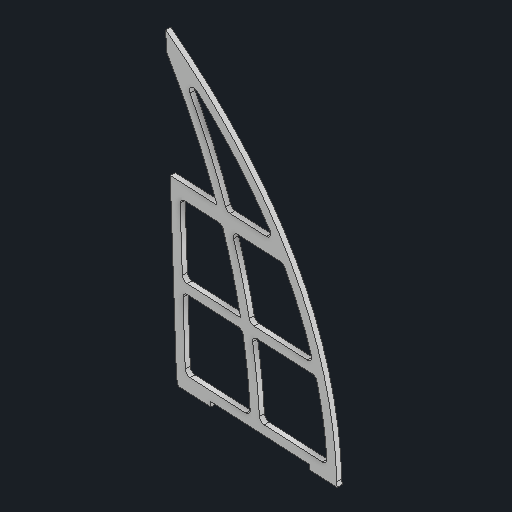
# Autodesk Inventor part: sponson_spanner_side
Saved by Autodesk Inventor 2023 (Build 270158030, 158C)
## iProperties
Created: 2022-03-22
Part Number: sponson_spanner_side
Material: Generic
Document SubType Name: Modeling
Designer: kardo
Density: 1 g/cm^3
Appearance: Default
Author: kardo
Autodesk Inventor part; units mm, degrees
ref_plane "YZ Plane" through (0, 0, 0) normal (1, 0, 0) x (0, 1, 0)
ref_plane "XZ Plane" through (0, 0, 0) normal (0, 1, 0) x (-1, 0, 0)
ref_plane "XY Plane" through (0, 0, 0) normal (0, 0, 1) x (1, 0, 0)
derived "surface_body.ipt"
sketch "sk_rail_sponson_side" plane through (81.12, 255, 36.448) normal (0.0461938, 0.0348622, -0.998324) x (0.2816917, -0.9592867, -0.0204648)
  line L0 (265.8225, 0) -> (150.1079, -34.011)
  spline S0 degree 2 poles (150.1079, -34.011) (71.6005, -57.0859) (0, 0) knots 0 0 0 1 1 1
  point P0 (222.5132, 151.1878)
ref_plane "plane_tunnel_right" through (81.12, 0, 0) normal (1, 0, 0) x (0, 1, 0)
ref_plane "plane_sponson_side" through (81.12, 255, 36.448) normal (0.0461938, 0.0348622, -0.998324) x (0.2816917, -0.9592867, -0.0204648)
sketch "sk_rail_sponson_tunnel" plane through (81.12, 0, 0) normal (1, 0, 0) x (0, 1, 0)
  line L0 (0, 0) -> (122.4, 8.559)
  line L1 (112.6461, 148.0459) -> (139.8617, -241.1549) construction
  spline S0 degree 2 poles (122.4, 8.559) (190.3044, 13.3074) (255, 36.448) knots 0 0 0 1 1 1
sketch "sk_rail_sponson_bottom" plane through (126.048, 0, 0) normal (0.3820078, -0.0644661, 0.9219079) x (-0.1718217, 0.9752166, 0.139391)
  line L0 (120.5596, -22.8124) -> (0, 0)
  line L1 (389.238, -73.6522) -> (-473.5511, 89.606) construction
  line L2 (163.9663, 206.5842) -> (90.6689, -180.7791) construction
  spline S0 degree 2 poles (120.5596, -22.8124) (192.7887, -36.4798) (261.4804, 0) knots 0 0 0 1 1 1
  point P0 (21.6578, 114.4574)
sketch "sk_rail_top_tunnel" plane through (81.12, 0, 0) normal (1, 0, 0) x (0, 1, 0)
  line L0 (255, 107.6209) -> (255, -224.5198) construction
  line L1 (0, 107.6209) -> (0, -224.5198) construction
  line L2 (-345, 107.6209) -> (-345, -224.5198) construction
  line L3 (-345, 0) -> (0, 0) construction
  line L4 (-172.5, 48.8998) -> (-172.5, 0) construction
  line L5 (0, 52.89) -> (37.026, 52.89) construction
  line L6 (37.026, 52.89) -> (80.784, 47.0555) construction
  line L7 (80.784, 47.0555) -> (112.2, 37.536) construction
  line L8 (112.2, 107.6209) -> (112.2, -224.5198) construction
  line L9 (0, 52.89) -> (255, 52.89) construction
  line L10 (-469.9272, 0) -> (379.2584, 0) construction
  spline S0 degree 3 poles (0, 52.89) (92.8353, 52.89) (195.0311, 49.5089) (255, 36.448) knots 0 0 0 0 1 1 1 1
  spline S1 degree 3 poles (0, 52.89) (37.026, 52.89) (80.784, 47.0555) (112.2, 37.536) knots 1 1 1 1 2 2 2 2
  spline S2 degree 4 poles (-345, 37.4554) (-258.8682, 45.1562) (-172.5926, 49.7838) (-86.3161, 52.89) (0, 52.89) knots 0 0 0 0 0 1 1 1 1 1
  point P0 (153, 48.7795)
  point P1 (112.2, 28.832)
  point P2 (-230.0001, 45.8702)
  point P3 (-114.9999, 51.0173)
sketch "sk_section_sponson_break" plane through (0, 122.4, 8.559) normal (0, 0.9975641, 0.0697565) x (-1, 0, 0)
  line L0 (-273.529, -60.9623) -> (62.2867, 77.8495) construction
  line L1 (-81.12, -262.9814) -> (-81.12, 151.9167) construction
  arc A0 (-81.12, 42.1186) -> (-156, 26.7233) centre (-71.3066, -195.4114) ccw construction
  arc A1 (-54.6, 54.2675) -> (-156, 30.9325) centre (-53.2768, -183.4615) ccw construction
  spline S0 degree 2 poles (-54.6, 54.2675) (-107.2974, 54.2675) (-156, 30.9325) knots 0 0 0 1 1 1
  spline S1 degree 2 poles (-156, 26.7233) (-120.0524, 40.429) (-81.12, 42.1186) knots 0 0 0 1 1 1
  point P0 (0, 0)
ref_plane "plane_sponson_break" through (0, 122.4, 8.559) normal (0, 0.9975641, 0.0697565) x (-1, 0, 0)
derived "parameters_frame.ipt"
derived "stencil_frame.ipt"
sketch "sk_joint_locations" plane through (81.12, 0, 0) normal (1, 0, 0) x (0, 1, 0)
  line L0 (0, 0) -> (122.4, 8.559) construction
  line L1 (36.465, 28.832) -> (112.2, 28.832) construction
  arc A0 (36.465, 28.832) -> (11.22, 28.376) centre (36.465, -670.197) ccw construction
  line L2 (-241.5001, 19.2432) -> (11.22, 28.376) construction
  line L3 (-345, 16.32) -> (-262.2001, 18.586) construction
  arc A1 (-262.2001, 18.586) -> (-241.5001, 19.2432) centre (-326.8578, 2381.2399) ccw construction
  line L4 (-95.1358, 3119.4657) -> (254.2444, -1876.9042) construction
  line L5 (-230.0001, 3089.1136) -> (-230.0001, -1866.0023) construction
  line L6 (-114.9999, 3089.1136) -> (-114.9999, -1866.0023) construction
  line L7 (-345, 3089.1136) -> (-345, -1866.0023) construction
  line L8 (0, 3089.1136) -> (0, -1866.0023) construction
  line L9 (516.4305, 45.5774) -> (-594.5903, 6.7797) construction
  line L10 (-657.7604, -27.3784) -> (621.8174, 62.0984) construction
  line L11 (193.4506, 30.2962) -> (193.1714, 38.2913) construction
  line L12 (201.1621, 36.7028) -> (201.7215, 28.7028) construction
  line L13 (0, 14.96) -> (121.9304, 15.2746) construction
  line L14 (-230.0001, 45.8702) -> (-230.0001, 19.6588) construction
  line L15 (-345, 37.4554) -> (-345, 16.32) construction
  line L16 (-114.9999, 51.0173) -> (-114.9999, 23.8147) construction
  line L17 (0, 52.89) -> (0, 27.9705) construction
  line L18 (119.462, 50.575) -> (119.9556, 43.5149) construction
  line L19 (120.4493, 36.4549) -> (119.9556, 43.5149) construction
  line L20 (120.4493, 36.4549) -> (120.943, 29.3948) construction
  line L21 (120.943, 29.3948) -> (121.4367, 22.3347) construction
  line L22 (121.4367, 22.3347) -> (121.9304, 15.2746) construction
  line L23 (0, 14.96) -> (0, 0) construction
  line L24 (112.2, 37.536) -> (112.2, 28.832) construction
  line L25 (112.2, 35.548) -> (112.2, 30.82) construction
  spline S0 degree 4 poles (-345, 37.4554) (-258.8682, 45.1562) (-172.5926, 49.7838) (-86.3161, 52.89) (0, 52.89) knots 0 0 0 0 0 1 1 1 1 1
  spline S1 degree 3 poles (0, 52.89) (92.8353, 52.89) (195.0311, 49.5089) (255, 36.448) knots 0 0 0 0 1 1 1 1
  spline S2 degree 2 poles (122.4, 8.559) (190.3044, 13.3074) (255, 36.448) knots 0 0 0 1 1 1
  point P0 (-95.1358, 3119.4657)
  point P1 (254.2444, -1876.9042)
  point P2 (193.311, 34.2938)
  point P3 (201.4418, 32.7028)
  point P4 (134.9575, 11.3411)
  point P5 (-345, 26.8877)
  point P6 (-230.0001, 32.7645)
  point P7 (-114.9999, 37.416)
  point P8 (0, 40.4303)
  point P9 (112.2, 33.184)
sketch "sk_spanner_joints_locations" plane through (0, 122.4, 8.559) normal (0, 0.9975641, 0.0697565) x (-1, 0, 0)
  line L0 (300.9234, 5.5808) -> (-420.7494, 38.9736) construction
  line L1 (-923.3057, -329.5522) -> (1264.6454, 574.8532) construction
  line L2 (-84.7099, 23.4246) -> (-83.6779, 17.514) construction
  line L3 (-84.7099, 23.4246) -> (-70.9223, 22.7866) construction
  line L4 (-83.6779, 17.514) -> (-70.9223, 22.7866) construction
  point P0 (0, 0)
  point P1 (-126.048, 0)
  point P2 (-156, 26.7233)
  point P3 (-141.742, 26.0635)
  point P4 (-98.9679, 24.0843)
  point P5 (-94.2704, 13.1355)
  point P6 (-115.4555, 4.3785)
ref_plane "plane_stringer_outer" through (84.12, 0, 0) normal (1, 0, 0) x (0, 1, 0)
sketch "sk_corner_offset" plane through (0, 122.4, 8.559) normal (0, 0.9975641, 0.0697565) x (-1, 0, 0)
  spline S0 degree 2 poles (-156, 26.7233) (-120.0524, 40.429) (-81.12, 42.1186) knots 0 0 0 1 1 1 construction
  line L0 (-156, 26.7233) -> (-126.048, 0) construction
  line L1 (-153.7218, 26.2989) -> (-125.2491, 0.8954) construction
  line L2 (-125.2491, 0.8954) -> (-126.048, 0) construction
  spline S1 degree 5 poles (-153.7218, 26.2988) (-139.7718, 31.4859) (-125.4179, 35.5876) (-110.7581, 38.5194) (-95.9372, 40.2742) (-81.068, 40.9197) knots 0 0 0 0 0 0 1 1 1 1 1 1 construction
  point P0 (0, 0)
  dimension "d9" = 1.2
  dimension "d10" = 1.2
  constraints: 6 end point, 1 coincident, 1 parallel, 1 perpendicular, 3 other
  measures "d10" distance between parallel lines of L1 L0
sketch "sk_tip_offset" plane through (81.12, 0, 0) normal (1, 0, 0) x (0, 1, 0)
  spline S0 degree 3 poles (0, 52.89) (92.8353, 52.89) (195.0311, 49.5089) (255, 36.448) knots 0 0 0 0 1 1 1 1 construction
  spline S1 degree 2 poles (122.4, 8.559) (190.3044, 13.3074) (255, 36.448) knots 0 0 0 1 1 1 construction
  spline S2 degree 5 poles (0, 51.69) (14.1108, 51.69) (28.2217, 51.6249) (42.3321, 51.4877) (70.2924, 51.0558) (98.2445, 50.2552) (112.0882, 49.7555) (138.5614, 48.5709) (165.0044, 46.8436) (177.6143, 45.8726) (199.84, 43.8477) (221.9828, 41.066) (231.553, 39.6839) (241.0942, 38.0879) (250.5671, 36.1558) knots 0 0 0 0 0 0 0.280662 0.280662 0.280662 0.556179 0.556179 0.556179 0.807705 0.807705 0.807705 1 1 1 1 1 1 construction
  spline S3 degree 5 poles (122.3163, 9.7561) (148.5177, 11.5885) (174.5986, 15.1479) (200.4027, 20.4751) (225.7629, 27.5171) (250.5671, 36.1559) knots 0 0 0 0 0 0 1 1 1 1 1 1 construction
  point P0 (0, 0)
  dimension "d7" = 1.2
  dimension "d8" = 1.2
  constraints: 1 coincident, 6 other
sketch "sk_sponson_spanner_side_base" plane through (81.12, 255, 36.448) normal (0.0461938, 0.0348622, -0.998324) x (0.2816917, -0.9592867, -0.0204648)
  spline S0 degree 2 poles (150.1079, -34.011) (71.6005, -57.0859) (0, 0) knots 0 0 0 1 1 1 construction
  line L0 (129.8727, 34.4266) -> (129.7052, 34.9929)
  line L1 (133.9197, 20.7391) -> (146.0609, -20.3235)
  line L2 (146.0609, -20.3235) -> (147.9788, -19.7564)
  line L3 (147.9788, -19.7564) -> (151.3759, -31.2458)
  line L4 (133.9197, 20.7391) -> (135.8376, 21.3061)
  line L5 (135.8376, 21.3061) -> (131.7906, 34.9936)
  line L6 (131.7906, 34.9936) -> (129.8727, 34.4266)
  line L7 (743.4792, 215.394) -> (-237.9642, -73.0729) projected
  line L8 (151.3759, -31.2458) -> (149.4464, -31.813)
  line L9 (265.8225, 0) -> (150.1079, -34.011) construction
  spline S1 degree 2 poles (4.2584, 1.2582) (73.4724, -54.1433) (149.4464, -31.813) knots 0 0 0 1 1 1
  point P0 (222.5132, 151.1878)
  point P1 (59.2215, 17.4064)
  point P2 (99.6986, 28.3676)
  point P3 (2.9008, -2.2776)
  point P4 (7.158, -1.0263)
  dimension "d3" = 2
  constraints: 16 end point, 4 parallel, 2 collinear, 2 perpendicular, 1 point on line, 3 other
  measures "d3" distance between parallel lines of L5 L1
extrude "thicken" add sketch "sk_sponson_spanner_side_base" along normal blind 2
sketch "sk_cut_weight" plane through (81.12, 255, 36.448) normal (0.0461938, 0.0348622, -0.998324) x (0.2816917, -0.9592867, -0.0204648)
  line L0 (129.8727, 34.4266) -> (129.7052, 34.9929) construction
  line L1 (133.9197, 20.7391) -> (146.0609, -20.3235) construction
  spline S0 degree 2 poles (4.2584, 1.2582) (73.4724, -54.1433) (149.4464, -31.813) knots 0 0 0 1 1 1 construction
  line L2 (59.2215, 17.4064) -> (73.1927, -30.1276) construction
  line L3 (65.034, 11.8154) -> (70.1822, -5.7002)
  line L4 (58.1495, 13.9611) -> (63.8883, -5.5639)
  line L5 (58.1495, 13.9611) -> (14.7215, 1.1967)
  line L6 (65.034, 11.8154) -> (127.0017, 30.029)
  line L7 (127.0017, 30.029) -> (135.0111, 2.9406)
  line L8 (71.3599, -9.707) -> (77.6679, -31.1685)
  line L9 (65.0759, -9.6042) -> (70.9366, -29.5438)
  line L10 (136.1454, -0.8957) -> (144.4717, -29.0561)
  line L11 (96.0179, 20.9222) -> (112.1912, -34.104) construction
  line L12 (101.2226, -3.8779) -> (94.099, 20.3582)
  line L13 (97.9367, 21.4862) -> (105.2323, -3.3355)
  line L14 (106.3717, -7.2119) -> (114.2458, -34.0018)
  line L15 (102.3649, -7.7644) -> (110.1278, -34.176)
  line L16 (743.4792, 215.394) -> (-237.9642, -73.0729) construction
  spline S1 degree 2 poles (139.9903, 0.2078) (75.0727, -18.9867) (7.158, -1.0263) knots 0 0 0 1 1 1
  spline S2 degree 5 poles (17.1654, -3.4748) (23.8169, -8.1942) (30.694, -12.5958) (37.8021, -16.6288) (53.8669, -24.5154) (70.9012, -30.0491) (80.4024, -32.2611) (99.0402, -34.8416) (117.8343, -34.1935) (126.8503, -33.1336) (135.7414, -31.3957) (144.4717, -29.0561) knots 0 0 0 0 0 0 0.303227 0.303227 0.303227 0.663954 0.663954 0.663954 1 1 1 1 1 1
  spline S3 degree 5 poles (135.0111, 2.9406) (123.1582, -0.3554) (111.0984, -2.907) (98.8829, -4.6588) (74.574, -6.4878) (50.2355, -5.1473) (38.2665, -3.7236) (26.4165, -1.5892) (14.7215, 1.1967) knots 0 0 0 0 0 0 0.505763 0.505763 0.505763 1 1 1 1 1 1
  point P0 (222.5132, 151.1878)
  dimension "d11" = 4
  dimension "d20" = 4
  dimension "d14" = 2
  dimension "d15" = 4
  dimension "d16" = 4
  dimension "d19" = 4
  dimension "d21" = 4
  constraints: 28 end point, 6 collinear, 5 parallel, 3 point on line, 2 midpoint, 2 perpendicular, 28 other
  measures "d14" distance between parallel lines of L2 L4
  measures "d15" distance between parallel lines of L2 L3
  measures "d16" distance between parallel lines of L1 L7
  measures "d19" distance between parallel lines of L13 L12
  measures "d21" distance between parallel lines of L16 L6
extrude "cut_weight" cut sketch "sk_cut_weight" along normal through all both and the other way through all contours L6 L12 S3 L3 | L6 L7 S3 L13 | L4 S3 L5 | S1 L15 S2 L8 | L9 S2 S1 | S1 L10 S2 L14
fillet "rounding" radius 2 18 edges at (88.1619, 124.7874, 31.225) (120.3757, 124.6834, 32.712) (117.4429, 159.0138, 33.7751) (88.1619, 159.061, 32.4219) (108.7022, 195.3002, 34.6378) (88.1619, 155.0634, 32.2823) (88.1619, 189.337, 33.4792) (110.5708, 189.3009, 34.5148) (89.3318, 239.5422, 35.2865) (118.042, 155.0152, 33.6632) (106.399, 189.3076, 34.322) (132.9162, 189.2648, 35.5475) (114.006, 155.0217, 33.4767) (145.9353, 154.9702, 34.9523) (129.463, 195.2667, 35.5973) (149.7098, 124.5888, 34.066) (144.9423, 158.9694, 35.046) (116.3794, 124.6963, 32.5275)
equation "\"d9\" = shell_thickness"
equation "\"d10\" = shell_thickness"
equation "\"d7\" = shell_thickness"
equation "\"d8\" = shell_thickness"
equation "\"d3\" = bulkhead_thickness"
equation "\"d5\" = bulkhead_thickness"
equation "\"d11\" = bulkhead_inset"
equation "\"d20\" = bulkhead_inset"
equation "\"d14\" = bulkhead_thickness"
equation "\"d15\" = 2 * bulkhead_thickness"
equation "\"d16\" = bulkhead_inset"
equation "\"d19\" = bulkhead_inset"
equation "\"d21\" = bulkhead_inset"
equation "\"d25\" = 0.5 * bulkhead_inset"
equation "\"d4\" = stringer_thickness"
equation "\"shell_thickness\" = 1.2"
equation "\"bulkhead_thickness\" = 2"
equation "\"bulkhead_inset\" = 4"
equation "\"stringer_thickness\" = 3"
body "Solid1"
